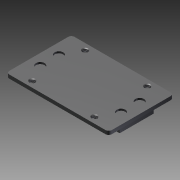
# Autodesk Inventor part: FBW2560R+640 L Slider
Saved by Autodesk Inventor 2011 SP1 (Build 150282100, 282)
## iProperties
Created: 2018-02-17
Part Number: FBW2560R+640 L Slider
Catalog Web Link: www.cadenas.de
Description: FBW2560RS-Satinless Steel Compact Type FBW2560XR
Vendor: THK
Document SubType Name: Modeling
Designer: psAdmin
Manufacturer: THK
Mass: 12.7162 g
Surface Area: 69.3459 cm^2
Volume: 12.7162 cm^3
Density: 1 g/cm^3
Category: PARTsolutions
Company: THK
Title: FBW2560R+640 L Slider
Author: Cadenas PARTsolutions
Comments: Satinless Steel Compact Type FBW2560XR
PSOL_IDENT_0: {$CADENAS_DATA\23d-libs\thk\linear_motion_systems\slide_pack\perpetual_lm_type_fbw\stainless_steel_c
PSOL_IDENT_1: ompact_type_fbw2560r\fbw_2560r_slider.prj},187 {VTYP=3D},{NB=FBW2560R+640 L Slider},{LINA=FBW2560R+6
PSOL_IDENT_2: 40 L Slider},{NN=FBW2560RS},{DATE=22.12.2017 01:25:51},{GEOMDATE=16.09.2015 01:22:00},{VERSION=},{LI
PSOL_IDENT_3: NEID=70},{LINESUBID=-1},{WBVAR=}  {NB=FBW2560R+640 L Slider},{LINA=FBW2560R+640 L Slider},{KT=DUMMY}
PSOL_IDENT_4: ,{IDNR=},{L=640},{N1=7},{G=40},{WOS=568},{WS=563},{M=290}
NN: FBW2560RS
NT: Satinless Steel Compact Type FBW2560XR
NB: FBW2560R+640 L Slider
NBSYN: FBW2560R+$L. L Slider
LINA: FBW2560R+640 L Slider
L: 640
N1: 7
G: 40
WOS: 568
WS: 563
M: 290
SUPPLIER: THK
ARTICLENO: FBW2560R+640 L Slider
BOMINFO: FBW2560R+640 L Slider
CREATOR: CADENAS GmbH
Autodesk Inventor part; units mm, degrees
sketch "Sketch_1" plane through (0, 0, 12) normal (0, 0, 1) x (1, 0, 0)
  arc A0 (0, -19) -> (2, -21) centre (2, -19) ccw
  line L0 (2, -21) -> (64, -21)
  arc A1 (64, -21) -> (66, -19) centre (64, -19) ccw
  line L1 (66, -19) -> (66, 19)
  arc A2 (66, 19) -> (64, 21) centre (64, 19) ccw
  line L2 (64, 21) -> (2, 21)
  arc A3 (2, 21) -> (0, 19) centre (2, 19) ccw
  line L3 (0, 19) -> (0, -19)
  constraints: 8 end point, 8 point on circle, 4 centre point
extrude "Extrusion1" add sketch "Sketch_1" against normal blind 2.3
sketch "Sketch_6" plane through (0, 0, 9.7) normal (0, 0, 1) x (1, 0, 0)
  line L0 (3, 10.9) -> (3, -10.9)
  line L1 (3, -10.9) -> (63, -10.9)
  line L2 (63, -10.9) -> (63, 10.9)
  line L3 (63, 10.9) -> (3, 10.9)
  constraints: 8 end point
extrude "Extrusion2" add sketch "Sketch_6" against normal blind 5
sketch "Sketch_2_ALT_Drilling_1" plane through (13, 0, 0) normal (1, 0, 0) x (0, 0, -1)
  line L0 (-12, 17) -> (-9.7, 17)
  line L1 (-9.7, 17) -> (-9.7, 15)
  line L2 (-9.7, 15) -> (-10.079, 15.379)
  line L3 (-10.079, 15.379) -> (-11.621, 15.379)
  line L4 (-11.621, 15.379) -> (-12, 15)
  line L5 (-12, 15) -> (-12, 17)
  line L6 (-12, 17) -> (-9.7, 17)
  constraints: 14 end point
revolve "Revolution1" cut sketch "Sketch_2_ALT_Drilling_1" angle 360 about axis through (13, 17, 12) along (0, 0, 1)
thread "Thread1" size "M4x0.7" class "6H" standard "ISO Metric profile" full length
sketch "Sketch_3_ALT_Drilling_2" plane through (13, 0, 0) normal (1, 0, 0) x (0, 0, -1)
  line L0 (-12, -17) -> (-9.7, -17)
  line L1 (-9.7, -17) -> (-9.7, -19)
  line L2 (-9.7, -19) -> (-10.079, -18.621)
  line L3 (-10.079, -18.621) -> (-11.621, -18.621)
  line L4 (-11.621, -18.621) -> (-12, -19)
  line L5 (-12, -19) -> (-12, -17)
  line L6 (-12, -17) -> (-9.7, -17)
  constraints: 14 end point
revolve "Revolution2" cut sketch "Sketch_3_ALT_Drilling_2" angle 360 about axis through (13, -17, 12) along (0, 0, 1)
thread "Thread2" size "M4x0.7" class "6H" standard "ISO Metric profile" full length
sketch "Sketch_4_ALT_Drilling_3" plane through (53, 0, 0) normal (1, 0, 0) x (0, 0, -1)
  line L0 (-12, 17) -> (-9.7, 17)
  line L1 (-9.7, 17) -> (-9.7, 15)
  line L2 (-9.7, 15) -> (-10.079, 15.379)
  line L3 (-10.079, 15.379) -> (-11.621, 15.379)
  line L4 (-11.621, 15.379) -> (-12, 15)
  line L5 (-12, 15) -> (-12, 17)
  line L6 (-12, 17) -> (-9.7, 17)
  constraints: 14 end point
revolve "Revolution3" cut sketch "Sketch_4_ALT_Drilling_3" angle 360 about axis through (53, 17, 12) along (0, 0, 1)
thread "Thread3" size "M4x0.7" class "6H" standard "ISO Metric profile" full length
sketch "Sketch_5_ALT_Drilling_4" plane through (53, 0, 0) normal (1, 0, 0) x (0, 0, -1)
  line L0 (-12, -17) -> (-9.7, -17)
  line L1 (-9.7, -17) -> (-9.7, -19)
  line L2 (-9.7, -19) -> (-10.079, -18.621)
  line L3 (-10.079, -18.621) -> (-11.621, -18.621)
  line L4 (-11.621, -18.621) -> (-12, -19)
  line L5 (-12, -19) -> (-12, -17)
  line L6 (-12, -17) -> (-9.7, -17)
  constraints: 14 end point
revolve "Revolution4" cut sketch "Sketch_5_ALT_Drilling_4" angle 360 about axis through (53, -17, 12) along (0, 0, 1)
thread "Thread4" size "M4x0.7" class "6H" standard "ISO Metric profile" full length
sketch "Sketch_8_ALT_Drilling_5" plane through (7, 0, 0) normal (1, 0, 0) x (0, 0, -1)
  line L0 (-10.85, 6) -> (-12, 6)
  line L1 (-12, 6) -> (-12, 8.75)
  line L2 (-12, 8.75) -> (-10.85, 8.75)
  line L3 (-10.85, 8.75) -> (-10.85, 6)
  line L4 (-10.85, 6) -> (-12, 6)
  constraints: 10 end point
revolve "Revolution5" cut sketch "Sketch_8_ALT_Drilling_5" angle 360 about axis through (7, 6, 10.85) along (0, 0, -1)
sketch "Sketch_9_ALT_Drilling_6" plane through (7, 0, 0) normal (1, 0, 0) x (0, 0, -1)
  line L0 (-10.85, -6) -> (-12, -6)
  line L1 (-12, -6) -> (-12, -3.25)
  line L2 (-12, -3.25) -> (-10.85, -3.25)
  line L3 (-10.85, -3.25) -> (-10.85, -6)
  line L4 (-10.85, -6) -> (-12, -6)
  constraints: 10 end point
revolve "Revolution6" cut sketch "Sketch_9_ALT_Drilling_6" angle 360 about axis through (7, -6, 10.85) along (0, 0, -1)
sketch "Sketch_10_ALT_Drilling_7" plane through (59, 0, 0) normal (1, 0, 0) x (0, 0, -1)
  line L0 (-10.85, 6) -> (-12, 6)
  line L1 (-12, 6) -> (-12, 8.75)
  line L2 (-12, 8.75) -> (-10.85, 8.75)
  line L3 (-10.85, 8.75) -> (-10.85, 6)
  line L4 (-10.85, 6) -> (-12, 6)
  constraints: 10 end point
revolve "Revolution7" cut sketch "Sketch_10_ALT_Drilling_7" angle 360 about axis through (59, 6, 10.85) along (0, 0, -1)
sketch "Sketch_11_ALT_Drilling_8" plane through (59, 0, 0) normal (1, 0, 0) x (0, 0, -1)
  line L0 (-10.85, -6) -> (-12, -6)
  line L1 (-12, -6) -> (-12, -3.25)
  line L2 (-12, -3.25) -> (-10.85, -3.25)
  line L3 (-10.85, -3.25) -> (-10.85, -6)
  line L4 (-10.85, -6) -> (-12, -6)
  constraints: 10 end point
revolve "Revolution8" cut sketch "Sketch_11_ALT_Drilling_8" angle 360 about axis through (59, -6, 10.85) along (0, 0, -1)
ref_plane "slider_ip1_XY" through (0, 0, 0) normal (1, 0, 0) x (0, 0, -1)
ref_plane "slider_ip1_YZ" through (0, 0, 0) normal (0, 0, -1) x (0, 1, 0)
ref_plane "slider_ip1_ZX" through (0, 0, 0) normal (0, 1, 0) x (1, 0, 0)
body "Solid1"
